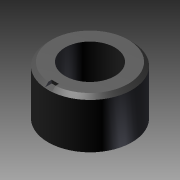
# Autodesk Inventor part: B12APbtoggl
Saved by Autodesk Inventor 2011 SP1 (Build 150282100, 282)
## iProperties
Created: 2013-12-24
Part Number: B12APbtoggl
Catalog Web Link: www.cadenas.de
Description: B Series - Body for Toggle-
Vendor: NKKSWITCHES
Document SubType Name: Modeling
Designer: PARTuser1
Manufacturer: NKKSWITCHES
Density: 1 g/cm^3
Category: PARTsolutions
Company: NKKSWITCHES
Title: B12APbtoggl
Author: Cadenas PARTsolutions
PSOL_IDENT_0: {$CADENAS_DATA\23d-libs\nkkswitches\toggle\b\parts\b_body_toggle.prj},215 {VTYP=3D},{NB=B12APbtoggl}
PSOL_IDENT_1: ,{LINA=B12APbtoggl},{NN=B Series - Body for Toggle},{DATE=06.03.2009 07:33:54},{GEOMDATE=27.02.2009
PSOL_IDENT_2: 11:41:00},{VERSION=},{LINEID=10},{LINESUBID=-1},{WBVAR=PLS,CRCTS,TGGLS,TRMNLS,CPS,CCLR}  {NB=B12APbt
PSOL_IDENT_3: oggl},{LINA=B12APbtoggl},{KT=DUMMY},{PN=B12AP},{SRS=B},{PLS=1},{CRCTS=2},{CRCTSALG= '2','2 - ON/NONE
PSOL_IDENT_4: /ON','3','3 - ON/OFF/ON','5','5 - ON/NONE/(ON)','R','R - (ON)/NONE/ON','8','8 - (ON)/OFF/(ON)','9','
PSOL_IDENT_5: 9 - ON/OFF/(ON)','S','S - (ON)/OFF/ON' },{TGGLS=A},{TGGLSALG=  'A','A - .394\" (10.0 mm) Bat','J','J
PSOL_IDENT_6: - .248\" (6.3 mm) Bat','E','E - .394\" (10.0 mm) Flatted','H','H - .248\" (6.3 mm) Flatted','K','K
PSOL_IDENT_7: - Snap Top for Paddles' },{TRMNLS=P},{TRMNLSALG= 'P','P - Straight','B','B - Straight with Bracket',
PSOL_IDENT_8: 'H','H - Right Angle with Bracket','V','V - Vertical with Bracket' ,'W','W - Straight Long' },{CPS=
PSOL_IDENT_9: },{CPSALG= '',' w/o Cap','G','G - .394\" (10.0 mm) Bat Lever Cap' },{CCLR=},{CCLR1= '', 'N/A' }
CNS_NN: B Series - Body for Toggle
CNS_NB: B12APbtoggl
CNS_NBSYN: $PN.btoggl
CNS_LINA: B12APbtoggl
CNS_PN: B12AP
CNS_SRS: B
CNS_PLS: 1 - SPDT
CNS_CRCTS: 2 - ON/NONE/ON
CNS_CRCTSALG: '2','2 - ON/NONE/ON','3','3 - ON/OFF/ON','5','5 - ON/NONE/(ON)','R','R - (ON)/NONE/ON','8','8 - (ON)/OFF/(ON)','9','9 - ON/OFF/(ON)','S','S - (ON)/OFF/ON'
CNS_TGGLS: A - .394" (10.0 mm) Bat
CNS_TGGLSALG: 'A','A - .394" (10.0 mm) Bat','J','J - .248" (6.3 mm) Bat','E','E - .394" (10.0 mm) Flatted','H','H - .248" (6.3 mm) Flatted','K','K - Snap Top for Paddles'
CNS_TRMNLS: P - Straight
CNS_TRMNLSALG: 'P','P - Straight','B','B - Straight with Bracket', 'H','H - Right Angle with Bracket','V','V - Vertical with Bracket' ,'W','W - Straight Long'
CNS_CPS: w/o Cap
CNS_CPSALG: '',' w/o Cap','G','G - .394" (10.0 mm) Bat Lever Cap'
CNS_CCLR: N/A
CNS_CCLR1: '', 'N/A'
SUPPLIER: NKKSWITCHES
ARTICLENO: B12APbtoggl
BOMINFO: B12APbtoggl
CREATOR: CADENAS GmbH
Autodesk Inventor part; units mm, degrees
sketch "Sketch_1" plane through (0, 0, 0) normal (1, 0, 0) x (0, 1, 0)
  line L0 (3.5052, 0) -> (0, 0)
  line L1 (0, 2.9972) -> (0, 1.778)
  line L2 (0, 1.778) -> (3.5052, 1.778)
  line L3 (3.5052, 1.778) -> (3.5052, 2.7432)
  line L4 (3.5052, 2.7432) -> (3.2512, 2.9972)
  line L5 (3.2512, 2.9972) -> (0, 2.9972)
  constraints: 12 end point
revolve "Revolution1" add sketch "Sketch_1" angle 360 about axis through (0, 3.5052, 0) along (0, 1, 0)
sketch "Sketch_10" plane through (0, 3.5052, 0) normal (0, 1, 0) x (1, 0, 0)
  line L0 (-0.254, -2.9972) -> (0.254, -2.9972)
  line L1 (0.254, -2.9972) -> (0.254, -2.4892)
  line L2 (0.254, -2.4892) -> (-0.254, -2.4892)
  line L3 (-0.254, -2.4892) -> (-0.254, -2.9972)
  constraints: 8 end point
extrude "Extrusion1" cut sketch "Sketch_10" against normal blind 0.2286
ref_plane "body_straight_XY" through (0, 0, 0) normal (0, 1, 0) x (1, 0, 0)
ref_plane "body_straight_YZ" through (0, 0, 0) normal (1, 0, 0) x (0, 0, -1)
ref_plane "body_straight_ZX" through (0, 0, 0) normal (0, 0, -1) x (0, 1, 0)
ref_plane "body_ver_ra_XY" through (0, 0, 0) normal (0, 0, 1) x (1, 0, 0)
ref_plane "body_ver_ra_YZ" through (0, 0, 0) normal (1, 0, 0) x (0, 1, 0)
ref_plane "body_ver_ra_ZX" through (0, 0, 0) normal (0, 1, 0) x (0, 0, 1)
ref_plane "cp_toggle__straight_XY" through (0, 3.5052, 0) normal (0, -1, 0) x (1, 0, 0)
ref_plane "cp_toggle__straight_YZ" through (0, 3.5052, 0) normal (1, 0, 0) x (0, 0, 1)
ref_plane "cp_toggle__straight_ZX" through (0, 3.5052, 0) normal (0, 0, 1) x (0, -1, 0)
ref_plane "toggle_vrtira_XY" through (0, 0, 3.5052) normal (0, 0, -1) x (1, 0, 0)
ref_plane "toggle_vrtira_YZ" through (0, 0, 3.5052) normal (1, 0, 0) x (0, -1, 0)
ref_plane "toggle_vrtira_ZX" through (0, 0, 3.5052) normal (0, -1, 0) x (0, 0, -1)
body "Solid1"
